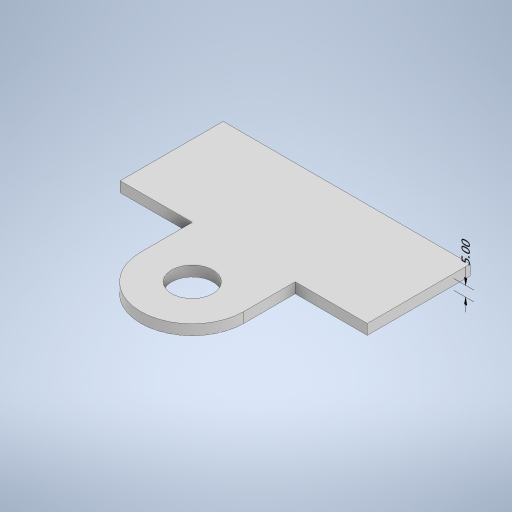
# Autodesk Inventor part: ギアプレート_ギアなし
Saved by Autodesk Inventor 2024.1 (Build 281209000, 209)
## iProperties
Created: 2024-04-01
Part Number: ギアプレート_ギアなし
Material: 一般
Document SubType Name: Modeling
Designer: hibik
Density: 1 g/cm^3
Appearance: 既定
Author: hibik
Autodesk Inventor part; units mm, degrees
ref_plane "YZ Plane" through (0, 0, 0) normal (1, 0, 0) x (0, 1, 0)
ref_plane "XZ Plane" through (0, 0, 0) normal (0, 1, 0) x (-1, 0, 0)
ref_plane "XY Plane" through (0, 0, 0) normal (0, 0, 1) x (1, 0, 0)
sketch "スケッチ1" plane through (0, 0, 0) normal (0, 1, 0) x (-1, 0, 0)
  line L0 (25, 0) -> (-25, 0)
  line L1 (-25, 0) -> (-25, -75)
  line L2 (-25, -75) -> (25, -75)
  line L3 (25, -75) -> (25, 0)
  circle A0 centre (0, 0) radius 25
  circle A1 centre (0, 0) radius 57 construction
  circle A2 centre (0, 0) radius 75 construction
  circle A3 centre (0, 0) radius 10
  dimension "d0" = 114
  dimension "d2" = 150
  dimension "d4" = 20
  dimension "d5" = 50
  constraints: 8 end point, 5 coincident, 4 centre point, 2 parallel, 2 tangent, 1 horizontal, 1 midpoint, 1 perpendicular
  measures "d0" diameter of A1
  measures "d2" diameter of A2
  measures "d4" diameter of A3
  measures "d5" distance of L1.end L2.end
extrude "押し出し1" add sketch "スケッチ1" along normal blind 5 contours A0 L0 A3 | L0 A3 A0 | L3 L2 L1 A0
sketch "スケッチ4" plane through (0, 5, 0) normal (0, 1, 0) x (1, 0, 0)
  line L0 (-60, 75) -> (60, 75)
  line L1 (60, 75) -> (60, 25)
  line L2 (60, 25) -> (-60, 25)
  line L3 (-60, 25) -> (-60, 75)
  line L4 (25, 75) -> (-25, 75) projected
  point P0 (0, 0)
  point P1 (0, 75)
  dimension "d24" = 50
  dimension "d25" = 120
  constraints: 8 end point, 2 midpoint, 2 parallel, 1 horizontal, 1 perpendicular
  measures "d24" distance of L0.end L1.end
  measures "d25" distance of L0.start L0.end
extrude "押し出し4" add sketch "スケッチ4" against normal up to surface (5 mm away)
